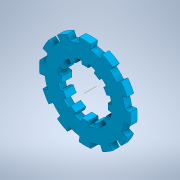
# Autodesk Inventor part: outerPartOfLock
Saved by Autodesk Inventor 2021.2 (Build 252289000, 289)
## iProperties
Created: 2020-11-07
Part Number: outerPartOfLock
Material: PC/ABS Plastic
Document SubType Name: Modeling
Designer: robst
Density: 0.357273 g/cm^3
Appearance: Sky Blue Medium
Author: robst
Autodesk Inventor part; units mm, degrees
ref_plane "YZ Plane" through (0, 0, 0) normal (1, 0, 0) x (0, 1, 0)
ref_plane "XZ Plane" through (0, 0, 0) normal (0, 1, 0) x (-1, 0, 0)
ref_plane "XY Plane" through (0, 0, 0) normal (0, 0, 1) x (1, 0, 0)
sketch "Sketch1" plane through (0, 0, 0) normal (0, 0, 1) x (1, 0, 0)
  circle A0 centre (0, 0) radius 38.1
  dimension "d0" = 76.2
  constraints: 1 centre point, 1 coincident
  measures "d0" diameter of A0
extrude "Extrusion1" add sketch "Sketch1" along normal mid plane 6.35
sketch "Sketch3" plane through (0, 0, 3.175) normal (0, 0, 1) x (1, 0, 0)
  circle A0 centre (0, 0) radius 25.4
  dimension "d8" = 50.8
  constraints: 1 centre point, 1 coincident
  measures "d8" diameter of A0
extrude "Extrusion3" cut sketch "Sketch3" against normal through all
sketch "Sketch4" plane through (0, 0, 3.175) normal (0, 0, 1) x (1, 0, 0)
  circle A0 centre (0, 0) radius 25.4 projected
  arc A1 (3.4556, 25.1638) -> (-3.175, 25.2008) centre (0, 0) ccw
  arc A2 (3.0033, 21.8699) -> (-2.7594, 21.902) centre (0, 0) ccw
  line L0 (3.0033, 21.8699) -> (3.4556, 25.1638)
  line L1 (-2.7594, 21.902) -> (-3.175, 25.2008)
  dimension "d32" = 3.3249
  dimension "d34" = 15
  constraints: 6 point on circle, 4 end point, 2 centre point, 2 coincident, 1 concentric
  measures "d32" radial gap between concentric circles of A2 A0
  measures "d34" angle of L0 L1
extrude "Extrusion8" add sketch "Sketch4" against normal blind 9.525 contours L0 A2 L1 A0 picked at (-2.3003, 24.1615)
pattern_circular "Circular Pattern3" count 12 over 360 about axis through (0, 0, -10) along (0, 0, 1) of "Extrusion8"
sketch "Sketch8" plane through (0, 0, 3.175) normal (0, 0, 1) x (1, 0, 0)
  arc A0 (5.624, 42.7187) -> (-5.624, 42.7187) centre (0, 0) ccw
  circle A1 centre (0, 0) radius 38.1 projected
  line L0 (4.973, 37.774) -> (5.624, 42.7187)
  line L1 (-4.973, 37.774) -> (-5.624, 42.7187)
  line L2 (0, 0) -> (0, 43.0873) construction
  arc A2 (4.973, 37.774) -> (-4.973, 37.774) centre (0, 0) ccw
  dimension "d40" = 4.9873
  dimension "d41" = 15
  dimension "d42" = 7.5
  constraints: 6 end point, 5 point on circle, 2 centre point, 2 coincident, 1 vertical
  measures "d40" radial gap between concentric circles of A1 A0
  measures "d41" angle of L0 L1
  measures "d42" angle of L1 L2
extrude "Extrusion9" add sketch "Sketch8" against normal blind 6.35 contours L0 A1 L1 A0
pattern_circular "Circular Pattern4" count 12 over 360 about axis through (0, 0, -10) along (0, 0, 1) of "Extrusion9"
equation "\"d0\" = externalDiameter"
equation "\"d8\" = internalDiameter"
equation "\"d32\" = depthOfInternalSpline"
equation "\"d35\" = thickness"
equation "\"d40\" = depthOfExternalSpline"
equation "\"internalDiameter\" = 50.8"
equation "\"externalDiameter\" = 76.2"
equation "\"pi\" = 3.141593"
equation "\"depthOfInternalSpline\" = 0.5 * widthOfInternalSpline"
equation "\"depthOfExternalSpline\" = 0.5 * widthOfExternalSpline"
equation "\"thickness\" = 9.525"
equation "\"widthOfInternalSpline\" = 6.649704"
equation "\"widthOfExternalSpline\" = 9.974557"
body "Solid1"
